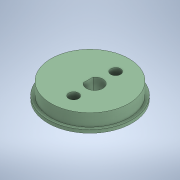
# Autodesk Inventor part: RotorShaft2
Saved by Autodesk Inventor 2021 (Build 250183000, 183)
## iProperties
Created: 2022-08-31
Part Number: RotorShaft2
Material: Ogólny
Document SubType Name: Modeling
Designer: MicnedSQ
Density: 1 g/cm^3
Appearance: Kauczuk — zielony
Author: MicnedSQ
Autodesk Inventor part; units mm, degrees
ref_plane "YZ Plane" through (0, 0, 0) normal (1, 0, 0) x (0, 1, 0)
ref_plane "XZ Plane" through (0, 0, 0) normal (0, 1, 0) x (-1, 0, 0)
ref_plane "XY Plane" through (0, 0, 0) normal (0, 0, 1) x (1, 0, 0)
sketch "Szkic1" plane through (0, 0, 0) normal (0, 1, 0) x (-1, 0, 0)
  circle A0 centre (0, 0) radius 13.5
  dimension "d0" = 27
  constraints: 1 centre point, 1 coincident
  measures "d0" diameter of A0
extrude "Wyciągnięcie proste1" add sketch "Szkic1" along normal blind 1
sketch "Szkic2" plane through (0, 1, 0) normal (0, 1, 0) x (1, 0, 0)
  circle A0 centre (0, 0) radius 12.5
  dimension "d3" = 25
  constraints: 1 centre point, 1 coincident
  measures "d3" diameter of A0
extrude "Wyciągnięcie proste2" add sketch "Szkic2" along normal blind 4
sketch "Szkic3" plane through (0, 5, 0) normal (0, 1, 0) x (1, 0, 0)
  point P0 (0, 0)
  point P1 (1.5, -6.75)
  point P2 (1.5, 6.75)
hole "Otwór1" at (1.5, 5, 6.75) at (1.5, 5, -6.75) direction (0, -1, 0) diameter 3.2 end through all
sketch "Szkic5" plane through (0, 0, 0) normal (0, -1, 0) x (1, 0, 0)
  arc A0 (-0.62, -1.59) -> (-0.62, 1.59) centre (1.5, 0) ccw
  line L0 (-0.62, 1.59) -> (-0.62, -1.59)
  point P0 (0, 0)
  dimension "d16" = 5.3
  constraints: 2 end point, 2 point on circle, 1 centre point, 1 vertical
  measures "d16" diameter of A0
extrude "Wyciągnięcie proste3" cut sketch "Szkic5" against normal through all
